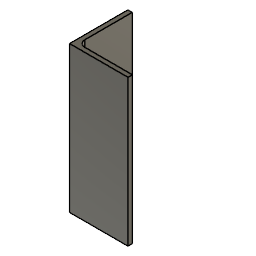
L-40×40×3 (Autodesk Fusion 360 design; units mm, degrees)
Autodesk Fusion 360 part; units mm, degrees
sketch "スケッチ1" plane through (0, 0, 0) normal (0, 0, 1) x (1, 0, 0)
  line L0 (40, 3) -> (7.5, 3)
  line L1 (0, 0) -> (40, 0)
  line L2 (0, 40) -> (0, 0)
  line L3 (3, 7.5) -> (3, 40)
  arc A0 (3, 7.5) -> (7.5, 3) centre (7.5, 7.5) ccw
  line L4 (3, 40) -> (0, 40)
  line L5 (40, 0) -> (40, 3)
extrude "押し出し1" add sketch "スケッチ1" along normal blind 100
